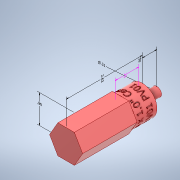
# Autodesk Inventor part: 1x8mmx1_1-inchHexShaft
Saved by Autodesk Inventor 2022.2 (Build 262287000, 287)
## iProperties
Created: 2020-11-16
Part Number: 1x8mmx1_1-inchHexShaft
Material: PC/ABS Plastic
Document SubType Name: Modeling
Designer: robst
Density: 0.357273 g/cm^3
Appearance: Smooth - Red
Author: robst
Autodesk Inventor part; units mm, degrees
ref_plane "XZ Plane" through (0, 0, 0) normal (0, 1, 0) x (-1, 0, 0)
ref_plane "XY Plane" through (0, 0, 0) normal (0, 0, 1) x (1, 0, 0)
sketch "Sketch1" plane through (0, 0, 0) normal (0, 0, 1) x (1, 0, 0)
  line L0 (14.6647, 0) -> (7.3323, -12.7)
  line L1 (7.3323, -12.7) -> (-7.3323, -12.7)
  line L2 (-7.3323, -12.7) -> (-14.6647, 0)
  line L3 (-14.6647, 0) -> (-7.3323, 12.7)
  line L4 (-7.3323, 12.7) -> (7.3323, 12.7)
  line L5 (7.3323, 12.7) -> (14.6647, 0)
  point P0 (0, 0)
  point P1 (0, 0)
  dimension "d0" = 25.4
  constraints: 12 end point, 1 coincident, 1 horizontal, 13 other
  measures "d0" distance between parallel lines of L1 L4
extrude "Hex Portion" add sketch "Sketch1" along normal mid plane 47.625
sketch "Sketch2" plane through (0, 0, -23.8125) normal (0, 0, -1) x (-1, 0, 0)
  circle A0 centre (0, 0) radius 12.7
  dimension "d3" = 25.4
  constraints: 1 centre point, 1 coincident
  measures "d3" diameter of A0
extrude "Extrusion2" add sketch "Sketch2" along normal blind 19.05
thicken "Reduce Size of Hex Shaft" operation add thickness 0.1905 both sides no extend neighbours yes toward (-0.8660254, -0.5, 0) faces at (10.9985, 6.35, 7.9375) (0, 12.7, 7.9375) (10.9985, -6.35, 7.9375) (0, -12.7, 7.9375) (-10.9985, -6.35, 7.9375) (-10.9985, 6.35, 7.9375)
sketch "Sketch3" plane through (0, 0, -42.8625) normal (0, 0, -1) x (-1, 0, 0)
  circle A0 centre (0, 0) radius 4
  dimension "d14" = 8
  constraints: 1 centre point, 1 coincident
  measures "d14" diameter of A0
extrude "Extrusion3" add sketch "Sketch3" along normal blind 12.7
ref_plane "Work Plane1" through (12.7, 0, -23.8125) normal (1, 0, 0) x (0, 1, 0)
sketch "Sketch4" plane through (12.7, 0, -23.8125) normal (1, 0, 0) x (0, 1, 0)
  line L0 (-12.7, 0) -> (12.7, 0) projected
  line L1 (-12.7, -19.05) -> (12.7, -19.05) projected
  line L2 (-12.7, 0) -> (-12.7, -19.05) construction
  line L3 (-12.7, -9.525) -> (12.7, -9.525) construction
  line L4 (12.7, 0) -> (12.7, -19.05) construction
  line L5 (-33.1661, -6.985) -> (-35.6444, -6.985)
  line L6 (-35.6444, -6.985) -> (-35.6444, -6.4663)
  line L7 (-35.6444, -6.4663) -> (-34.7223, -6.4663)
  line L8 (-34.7223, -6.4663) -> (-34.7223, -3.0618)
  line L9 (-34.7223, -3.0618) -> (-35.6444, -3.0618)
  line L10 (-35.6444, -3.0618) -> (-35.6444, -2.5966)
  spline S0 degree 2 poles (-35.6444, -2.5966) (-35.1216, -2.5966) (-34.6276, -2.3002) (-34.5946, -1.8885) knots 0 0 0 1 2 2 2
  line L11 (-34.5946, -1.8885) -> (-34.0677, -1.8885)
  line L12 (-34.0677, -1.8885) -> (-34.0677, -6.4663)
  line L13 (-34.0677, -6.4663) -> (-33.1661, -6.4663)
  line L14 (-33.1661, -6.4663) -> (-33.1661, -6.985)
  line L15 (-31.4701, -1.6786) -> (-31.6183, -3.6546)
  line L16 (-31.6183, -3.6546) -> (-32.067, -3.6546)
  line L17 (-32.067, -3.6546) -> (-32.2152, -1.6786)
  line L18 (-32.2152, -1.6786) -> (-31.4701, -1.6786)
  line L19 (-30.1857, -1.6786) -> (-30.3339, -3.6546)
  line L20 (-30.3339, -3.6546) -> (-30.7826, -3.6546)
  line L21 (-30.7826, -3.6546) -> (-30.9308, -1.6786)
  line L22 (-30.9308, -1.6786) -> (-30.1857, -1.6786)
  line L23 (-24.1918, -6.985) -> (-24.978, -6.985)
  line L24 (-24.978, -6.985) -> (-25.9043, -5.5524)
  line L25 (-25.9043, -5.5524) -> (-26.8553, -6.985)
  line L26 (-26.8553, -6.985) -> (-27.5839, -6.985)
  line L27 (-27.5839, -6.985) -> (-26.2624, -5.0954)
  line L28 (-26.2624, -5.0954) -> (-27.5716, -3.1729)
  line L29 (-27.5716, -3.1729) -> (-26.7853, -3.1729)
  line L30 (-26.7853, -3.1729) -> (-25.8631, -4.5932)
  line L31 (-25.8631, -4.5932) -> (-24.9204, -3.1729)
  line L32 (-24.9204, -3.1729) -> (-24.1918, -3.1729)
  line L33 (-24.1918, -3.1729) -> (-25.505, -5.0543)
  line L34 (-25.505, -5.0543) -> (-24.1918, -6.985)
  spline S1 degree 2 poles (-20.0709, -7.1003) (-20.4497, -7.1003) (-21.0713, -6.8738) (-21.2895, -6.6639) knots 0 0 0 1 2 2 2
  spline S2 degree 2 poles (-21.2895, -6.6639) (-21.5036, -6.4581) (-21.7259, -5.8982) (-21.7259, -5.5812) knots 0 0 0 1 2 2 2
  spline S3 degree 2 poles (-21.7259, -5.5812) (-21.7259, -5.1695) (-21.2854, -4.4779) (-20.8655, -4.2721) knots 0 0 0 1 2 2 2
  line L35 (-20.8655, -4.2721) -> (-20.8655, -4.2515)
  spline S4 degree 2 poles (-20.8655, -4.2515) (-21.2401, -4.0333) (-21.6024, -3.5146) (-21.6024, -3.1277) knots 0 0 0 1 2 2 2
  spline S5 degree 2 poles (-21.6024, -3.1277) (-21.6024, -2.5554) (-20.7378, -1.7897) (-20.0709, -1.7897) knots 0 0 0 1 2 2 2
  spline S6 degree 2 poles (-20.0709, -1.7897) (-19.3793, -1.7897) (-18.5436, -2.5143) (-18.5436, -3.0824) knots 0 0 0 1 2 2 2
  spline S7 degree 2 poles (-18.5436, -3.0824) (-18.5436, -3.4241) (-18.943, -4.091) (-19.3176, -4.2803) knots 0 0 0 1 2 2 2
  line L36 (-19.3176, -4.2803) -> (-19.3176, -4.3009)
  spline S8 degree 2 poles (-19.3176, -4.3009) (-18.873, -4.5068) (-18.416, -5.0996) (-18.416, -5.5689) knots 0 0 0 1 2 2 2
  spline S9 degree 2 poles (-18.416, -5.5689) (-18.416, -6.2193) (-19.3629, -7.1003) (-20.0709, -7.1003) knots 0 0 0 1 2 2 2
  spline S10 degree 2 poles (-19.1159, -5.6347) (-19.1159, -5.3219) (-19.3629, -4.9514) (-19.7128, -4.762) knots 0 0 0 1 2 2 2
  spline S11 degree 2 poles (-19.7128, -4.762) (-19.8281, -4.6961) (-20.215, -4.5438) (-20.4579, -4.445) knots 0 0 0 1 2 2 2
  spline S12 degree 2 poles (-20.4579, -4.445) (-20.7378, -4.6303) (-21.0384, -5.1819) (-21.0384, -5.5318) knots 0 0 0 1 2 2 2
  spline S13 degree 2 poles (-21.0384, -5.5318) (-21.0384, -5.9929) (-20.4826, -6.5939) (-20.0627, -6.5939) knots 0 0 0 1 2 2 2
  spline S14 degree 2 poles (-20.0627, -6.5939) (-19.6346, -6.5939) (-19.1159, -6.0793) (-19.1159, -5.6347) knots 0 0 0 1 2 2 2
  spline S15 degree 2 poles (-19.2106, -3.0906) (-19.2106, -2.7489) (-19.6675, -2.292) (-20.0751, -2.292) knots 0 0 0 1 2 2 2
  spline S16 degree 2 poles (-20.0751, -2.292) (-20.4456, -2.292) (-20.919, -2.6995) (-20.919, -3.0494) knots 0 0 0 1 2 2 2
  spline S17 degree 2 poles (-20.919, -3.0494) (-20.919, -3.3006) (-20.6761, -3.6505) (-20.4332, -3.7904) knots 0 0 0 1 2 2 2
  spline S18 degree 2 poles (-20.4332, -3.7904) (-20.3303, -3.8481) (-19.8939, -4.0498) (-19.7169, -4.1074) knots 0 0 0 1 2 2 2
  spline S19 degree 2 poles (-19.7169, -4.1074) (-19.4205, -3.881) (-19.2106, -3.3994) (-19.2106, -3.0906) knots 0 0 0 1 2 2 2
  line L37 (-13.3772, -6.985) -> (-13.3772, -4.7785)
  spline S20 degree 2 poles (-13.3772, -4.7785) (-13.3772, -4.515) (-13.4184, -4.0663) (-13.4842, -3.9428) knots 0 0 0 1 2 2 2
  spline S21 degree 2 poles (-13.4842, -3.9428) (-13.5501, -3.8069) (-13.8012, -3.6752) (-14.0194, -3.6752) knots 0 0 0 1 2 2 2
  spline S22 degree 2 poles (-14.0194, -3.6752) (-14.217, -3.6752) (-14.6698, -3.9181) (-14.9086, -4.1486) knots 0 0 0 1 2 2 2
  spline S23 degree 2 poles (-14.9086, -4.1486) (-14.9045, -4.2062) (-14.8963, -4.3668) (-14.8963, -4.4738) knots 0 0 0 1 2 2 2
  line L38 (-14.8963, -4.4738) -> (-14.8963, -6.985)
  line L39 (-14.8963, -6.985) -> (-15.5385, -6.985)
  line L40 (-15.5385, -6.985) -> (-15.5385, -4.7785)
  spline S24 degree 2 poles (-15.5385, -4.7785) (-15.5385, -4.515) (-15.5796, -4.0663) (-15.6455, -3.9428) knots 0 0 0 1 2 2 2
  spline S25 degree 2 poles (-15.6455, -3.9428) (-15.7114, -3.8069) (-15.9625, -3.6752) (-16.1807, -3.6752) knots 0 0 0 1 2 2 2
  spline S26 degree 2 poles (-16.1807, -3.6752) (-16.3865, -3.6752) (-16.8435, -3.9345) (-17.0575, -4.1362) knots 0 0 0 1 2 2 2
  line L41 (-17.0575, -4.1362) -> (-17.0575, -6.985)
  line L42 (-17.0575, -6.985) -> (-17.6997, -6.985)
  line L43 (-17.6997, -6.985) -> (-17.6997, -3.1729)
  line L44 (-17.6997, -3.1729) -> (-17.0575, -3.1729)
  line L45 (-17.0575, -3.1729) -> (-17.0575, -3.5928)
  spline S27 degree 2 poles (-17.0575, -3.5928) (-16.8064, -3.3417) (-16.3124, -3.0659) (-16.016, -3.0659) knots 0 0 0 1 2 2 2
  spline S28 degree 2 poles (-16.016, -3.0659) (-15.6784, -3.0659) (-15.1556, -3.3747) (-15.0198, -3.7246) knots 0 0 0 1 2 2 2
  spline S29 degree 2 poles (-15.0198, -3.7246) (-14.7275, -3.3994) (-14.1758, -3.0659) (-13.8547, -3.0659) knots 0 0 0 1 2 2 2
  spline S30 degree 2 poles (-13.8547, -3.0659) (-13.6077, -3.0659) (-13.2043, -3.2182) (-13.0561, -3.3911) knots 0 0 0 1 2 2 2
  spline S31 degree 2 poles (-13.0561, -3.3911) (-12.9038, -3.564) (-12.735, -4.0827) (-12.735, -4.4738) knots 0 0 0 1 2 2 2
  line L46 (-12.735, -4.4738) -> (-12.735, -6.985)
  line L47 (-12.735, -6.985) -> (-13.3772, -6.985)
  line L48 (-7.5109, -6.985) -> (-7.5109, -4.7785)
  spline S32 degree 2 poles (-7.5109, -4.7785) (-7.5109, -4.515) (-7.5521, -4.0663) (-7.6179, -3.9428) knots 0 0 0 1 2 2 2
  spline S33 degree 2 poles (-7.6179, -3.9428) (-7.6838, -3.8069) (-7.9349, -3.6752) (-8.1531, -3.6752) knots 0 0 0 1 2 2 2
  spline S34 degree 2 poles (-8.1531, -3.6752) (-8.3507, -3.6752) (-8.8036, -3.9181) (-9.0423, -4.1486) knots 0 0 0 1 2 2 2
  spline S35 degree 2 poles (-9.0423, -4.1486) (-9.0382, -4.2062) (-9.03, -4.3668) (-9.03, -4.4738) knots 0 0 0 1 2 2 2
  line L49 (-9.03, -4.4738) -> (-9.03, -6.985)
  line L50 (-9.03, -6.985) -> (-9.6722, -6.985)
  line L51 (-9.6722, -6.985) -> (-9.6722, -4.7785)
  spline S36 degree 2 poles (-9.6722, -4.7785) (-9.6722, -4.515) (-9.7133, -4.0663) (-9.7792, -3.9428) knots 0 0 0 1 2 2 2
  spline S37 degree 2 poles (-9.7792, -3.9428) (-9.8451, -3.8069) (-10.0962, -3.6752) (-10.3144, -3.6752) knots 0 0 0 1 2 2 2
  spline S38 degree 2 poles (-10.3144, -3.6752) (-10.5202, -3.6752) (-10.9772, -3.9345) (-11.1912, -4.1362) knots 0 0 0 1 2 2 2
  line L52 (-11.1912, -4.1362) -> (-11.1912, -6.985)
  line L53 (-11.1912, -6.985) -> (-11.8334, -6.985)
  line L54 (-11.8334, -6.985) -> (-11.8334, -3.1729)
  line L55 (-11.8334, -3.1729) -> (-11.1912, -3.1729)
  line L56 (-11.1912, -3.1729) -> (-11.1912, -3.5928)
  spline S39 degree 2 poles (-11.1912, -3.5928) (-10.9401, -3.3417) (-10.4461, -3.0659) (-10.1497, -3.0659) knots 0 0 0 1 2 2 2
  spline S40 degree 2 poles (-10.1497, -3.0659) (-9.8121, -3.0659) (-9.2893, -3.3747) (-9.1535, -3.7246) knots 0 0 0 1 2 2 2
  spline S41 degree 2 poles (-9.1535, -3.7246) (-8.8612, -3.3994) (-8.3095, -3.0659) (-7.9884, -3.0659) knots 0 0 0 1 2 2 2
  spline S42 degree 2 poles (-7.9884, -3.0659) (-7.7414, -3.0659) (-7.338, -3.2182) (-7.1898, -3.3911) knots 0 0 0 1 2 2 2
  spline S43 degree 2 poles (-7.1898, -3.3911) (-7.0375, -3.564) (-6.8687, -4.0827) (-6.8687, -4.4738) knots 0 0 0 1 2 2 2
  line L57 (-6.8687, -4.4738) -> (-6.8687, -6.985)
  line L58 (-6.8687, -6.985) -> (-7.5109, -6.985)
  line L59 (-0.8254, -6.985) -> (-1.6117, -6.985)
  line L60 (-1.6117, -6.985) -> (-2.5379, -5.5524)
  line L61 (-2.5379, -5.5524) -> (-3.4889, -6.985)
  line L62 (-3.4889, -6.985) -> (-4.2176, -6.985)
  line L63 (-4.2176, -6.985) -> (-2.8961, -5.0954)
  line L64 (-2.8961, -5.0954) -> (-4.2052, -3.1729)
  line L65 (-4.2052, -3.1729) -> (-3.4189, -3.1729)
  line L66 (-3.4189, -3.1729) -> (-2.4968, -4.5932)
  line L67 (-2.4968, -4.5932) -> (-1.5541, -3.1729)
  line L68 (-1.5541, -3.1729) -> (-0.8254, -3.1729)
  line L69 (-0.8254, -3.1729) -> (-2.1386, -5.0543)
  line L70 (-2.1386, -5.0543) -> (-0.8254, -6.985)
  line L71 (4.6375, -6.985) -> (2.1592, -6.985)
  line L72 (2.1592, -6.985) -> (2.1592, -6.4663)
  line L73 (2.1592, -6.4663) -> (3.0813, -6.4663)
  line L74 (3.0813, -6.4663) -> (3.0813, -3.0618)
  line L75 (3.0813, -3.0618) -> (2.1592, -3.0618)
  line L76 (2.1592, -3.0618) -> (2.1592, -2.5966)
  spline S44 degree 2 poles (2.1592, -2.5966) (2.682, -2.5966) (3.176, -2.3002) (3.209, -1.8885) knots 0 0 0 1 2 2 2
  line L77 (3.209, -1.8885) -> (3.7359, -1.8885)
  line L78 (3.7359, -1.8885) -> (3.7359, -6.4663)
  line L79 (3.7359, -6.4663) -> (4.6375, -6.4663)
  line L80 (4.6375, -6.4663) -> (4.6375, -6.985)
  line L81 (6.6629, -6.985) -> (5.8478, -6.985)
  line L82 (5.8478, -6.985) -> (5.8478, -6.0135)
  line L83 (5.8478, -6.0135) -> (6.6629, -6.0135)
  line L84 (6.6629, -6.0135) -> (6.6629, -6.985)
  spline S45 degree 2 poles (10.8495, -4.445) (10.8495, -5.8117) (10.055, -7.092) (9.2276, -7.092) knots 0 0 0 1 2 2 2
  spline S46 degree 2 poles (9.2276, -7.092) (8.3878, -7.092) (7.6015, -5.787) (7.6015, -4.4491) knots 0 0 0 1 2 2 2
  spline S47 degree 2 poles (7.6015, -4.4491) (7.6015, -3.0741) (8.396, -1.8021) (9.2276, -1.8021) knots 0 0 0 1 2 2 2
  spline S48 degree 2 poles (9.2276, -1.8021) (10.0633, -1.8021) (10.8495, -3.1194) (10.8495, -4.445) knots 0 0 0 1 2 2 2
  spline S49 degree 2 poles (9.9768, -5.9929) (10.0756, -5.7418) (10.1579, -4.9678) (10.1579, -4.445) knots 0 0 0 1 2 2 2
  spline S50 degree 2 poles (10.1579, -4.445) (10.1579, -3.9222) (10.0756, -3.1524) (9.9727, -2.893) knots 0 0 0 1 2 2 2
  spline S51 degree 2 poles (9.9727, -2.893) (9.8698, -2.6337) (9.5116, -2.3661) (9.2276, -2.3661) knots 0 0 0 1 2 2 2
  spline S52 degree 2 poles (9.2276, -2.3661) (8.9435, -2.3661) (8.5771, -2.6337) (8.4701, -2.9012) knots 0 0 0 1 2 2 2
  spline S53 degree 2 poles (8.4701, -2.9012) (8.3672, -3.1606) (8.2931, -3.951) (8.2931, -4.4491) knots 0 0 0 1 2 2 2
  spline S54 degree 2 poles (8.2931, -4.4491) (8.2931, -4.9843) (8.3589, -5.7006) (8.466, -5.9805) knots 0 0 0 1 2 2 2
  spline S55 degree 2 poles (8.466, -5.9805) (8.5648, -6.244) (8.9312, -6.528) (9.2276, -6.528) knots 0 0 0 1 2 2 2
  spline S56 degree 2 poles (9.2276, -6.528) (9.5075, -6.528) (9.8739, -6.2605) (9.9768, -5.9929) knots 0 0 0 1 2 2 2
  line L85 (12.2616, -1.6786) -> (12.1134, -3.6546)
  line L86 (12.1134, -3.6546) -> (11.6647, -3.6546)
  line L87 (11.6647, -3.6546) -> (11.5164, -1.6786)
  line L88 (11.5164, -1.6786) -> (12.2616, -1.6786)
  line L89 (13.546, -1.6786) -> (13.3978, -3.6546)
  line L90 (13.3978, -3.6546) -> (12.9491, -3.6546)
  line L91 (12.9491, -3.6546) -> (12.8009, -1.6786)
  line L92 (12.8009, -1.6786) -> (13.546, -1.6786)
  spline S57 degree 2 poles (18.6136, -7.0756) (18.1196, -7.0756) (17.2839, -6.7421) (16.9793, -6.4087) knots 0 0 0 1 2 2 2
  spline S58 degree 2 poles (16.9793, -6.4087) (16.6747, -6.0793) (16.3412, -5.0913) (16.3412, -4.4491) knots 0 0 0 1 2 2 2
  spline S59 degree 2 poles (16.3412, -4.4491) (16.3412, -3.811) (16.6664, -2.8642) (16.9752, -2.5143) knots 0 0 0 1 2 2 2
  spline S60 degree 2 poles (16.9752, -2.5143) (17.2798, -2.1726) (18.1114, -1.8144) (18.626, -1.8144) knots 0 0 0 1 2 2 2
  spline S61 degree 2 poles (18.626, -1.8144) (18.8812, -1.8144) (19.3299, -1.8885) (19.5193, -1.9462) knots 0 0 0 1 2 2 2
  spline S62 degree 2 poles (19.5193, -1.9462) (19.684, -1.9997) (20.0257, -2.152) (20.1944, -2.2426) knots 0 0 0 1 2 2 2
  line L93 (20.1944, -2.2426) -> (20.1944, -3.0577)
  line L94 (20.1944, -3.0577) -> (20.1409, -3.0577)
  spline S63 degree 2 poles (20.1409, -3.0577) (20.0504, -2.9753) (19.7704, -2.7448) (19.5687, -2.6337) knots 0 0 0 1 2 2 2
  spline S64 degree 2 poles (19.5687, -2.6337) (19.3752, -2.5266) (18.9183, -2.3908) (18.6219, -2.3908) knots 0 0 0 1 2 2 2
  spline S65 degree 2 poles (18.6219, -2.3908) (18.2966, -2.3908) (17.7162, -2.6584) (17.498, -2.9136) knots 0 0 0 1 2 2 2
  spline S66 degree 2 poles (17.498, -2.9136) (17.2839, -3.1729) (17.0452, -3.9592) (17.0452, -4.4491) knots 0 0 0 1 2 2 2
  spline S67 degree 2 poles (17.0452, -4.4491) (17.0452, -4.9719) (17.2963, -5.7253) (17.5145, -5.9846) knots 0 0 0 1 2 2 2
  spline S68 degree 2 poles (17.5145, -5.9846) (17.7285, -6.2358) (18.3008, -6.491) (18.6219, -6.491) knots 0 0 0 1 2 2 2
  spline S69 degree 2 poles (18.6219, -6.491) (18.9141, -6.491) (19.4123, -6.3469) (19.6058, -6.2399) knots 0 0 0 1 2 2 2
  spline S70 degree 2 poles (19.6058, -6.2399) (19.791, -6.1328) (20.0668, -5.9105) (20.145, -5.8323) knots 0 0 0 1 2 2 2
  line L95 (20.145, -5.8323) -> (20.1944, -5.8323)
  line L96 (20.1944, -5.8323) -> (20.1944, -6.6392)
  spline S71 degree 2 poles (20.1944, -6.6392) (20.0257, -6.7174) (19.7293, -6.8615) (19.5193, -6.9274) knots 0 0 0 1 2 2 2
  spline S72 degree 2 poles (19.5193, -6.9274) (19.297, -7.0015) (18.9183, -7.0756) (18.6136, -7.0756) knots 0 0 0 1 2 2 2
  spline S73 degree 2 poles (22.4298, -7.0715) (21.5159, -7.0715) (20.5114, -6.0464) (20.5114, -5.0996) knots 0 0 0 1 2 2 2
  spline S74 degree 2 poles (20.5114, -5.0996) (20.5114, -4.1692) (21.4871, -3.0659) (22.2734, -3.0659) knots 0 0 0 1 2 2 2
  spline S75 degree 2 poles (22.2734, -3.0659) (22.6274, -3.0659) (23.1749, -3.2717) (23.3766, -3.4899) knots 0 0 0 1 2 2 2
  spline S76 degree 2 poles (23.3766, -3.4899) (23.5825, -3.7081) (23.8007, -4.338) (23.8007, -4.7949) knots 0 0 0 1 2 2 2
  line L97 (23.8007, -4.7949) -> (23.8007, -5.1448)
  line L98 (23.8007, -5.1448) -> (21.1619, -5.1448)
  spline S77 degree 2 poles (21.1619, -5.1448) (21.1619, -5.8076) (21.8288, -6.5116) (22.4216, -6.5116) knots 0 0 0 1 2 2 2
  spline S78 degree 2 poles (22.4216, -6.5116) (22.6315, -6.5116) (23.0391, -6.4169) (23.2037, -6.3428) knots 0 0 0 1 2 2 2
  spline S79 degree 2 poles (23.2037, -6.3428) (23.3766, -6.2605) (23.6154, -6.1164) (23.6936, -6.0505) knots 0 0 0 1 2 2 2
  line L99 (23.6936, -6.0505) -> (23.7307, -6.0505)
  line L100 (23.7307, -6.0505) -> (23.7307, -6.7503)
  spline S80 degree 2 poles (23.7307, -6.7503) (23.6195, -6.7956) (23.282, -6.9274) (23.1502, -6.9644) knots 0 0 0 1 2 2 2
  spline S81 degree 2 poles (23.1502, -6.9644) (22.965, -7.0179) (22.6603, -7.0715) (22.4298, -7.0715) knots 0 0 0 1 2 2 2
  spline S82 degree 2 poles (23.1749, -4.655) (23.1667, -4.3956) (23.0597, -4.0169) (22.9567, -3.8892) knots 0 0 0 1 2 2 2
  spline S83 degree 2 poles (22.9567, -3.8892) (22.8456, -3.7452) (22.4957, -3.5928) (22.2363, -3.5928) knots 0 0 0 1 2 2 2
  spline S84 degree 2 poles (22.2363, -3.5928) (21.9811, -3.5928) (21.6229, -3.7452) (21.4747, -3.8934) knots 0 0 0 1 2 2 2
  spline S85 degree 2 poles (21.4747, -3.8934) (21.3306, -4.0457) (21.1824, -4.4121) (21.1619, -4.655) knots 0 0 0 1 2 2 2
  line L101 (21.1619, -4.655) -> (23.1749, -4.655)
  line L102 (27.4439, -6.985) -> (26.8017, -6.985)
  line L103 (26.8017, -6.985) -> (26.8017, -4.8114)
  spline S86 degree 2 poles (26.8017, -4.8114) (26.8017, -4.5479) (26.7523, -4.0951) (26.6782, -3.9592) knots 0 0 0 1 2 2 2
  spline S87 degree 2 poles (26.6782, -3.9592) (26.6, -3.8151) (26.3201, -3.6752) (26.0813, -3.6752) knots 0 0 0 1 2 2 2
  spline S88 degree 2 poles (26.0813, -3.6752) (25.8425, -3.6752) (25.3362, -3.9304) (25.0933, -4.1362) knots 0 0 0 1 2 2 2
  line L104 (25.0933, -4.1362) -> (25.0933, -6.985)
  line L105 (25.0933, -6.985) -> (24.4511, -6.985)
  line L106 (24.4511, -6.985) -> (24.4511, -3.1729)
  line L107 (24.4511, -3.1729) -> (25.0933, -3.1729)
  line L108 (25.0933, -3.1729) -> (25.0933, -3.597)
  spline S89 degree 2 poles (25.0933, -3.597) (25.3815, -3.3376) (25.9372, -3.0659) (26.2501, -3.0659) knots 0 0 0 1 2 2 2
  spline S90 degree 2 poles (26.2501, -3.0659) (26.81, -3.0659) (27.4439, -3.8069) (27.4439, -4.5109) knots 0 0 0 1 2 2 2
  line L109 (27.4439, -4.5109) -> (27.4439, -6.985)
  spline S91 degree 2 poles (29.4982, -7.0591) (28.9753, -7.0591) (28.3867, -6.4622) (28.3867, -5.8159) knots 0 0 0 1 2 2 2
  line L110 (28.3867, -5.8159) -> (28.3867, -3.704)
  line L111 (28.3867, -3.704) -> (27.9544, -3.704)
  line L112 (27.9544, -3.704) -> (27.9544, -3.1729)
  line L113 (27.9544, -3.1729) -> (28.3867, -3.1729)
  line L114 (28.3867, -3.1729) -> (28.3867, -2.0779)
  line L115 (28.3867, -2.0779) -> (29.0289, -2.0779)
  line L116 (29.0289, -2.0779) -> (29.0289, -3.1729)
  line L117 (29.0289, -3.1729) -> (30.2104, -3.1729)
  line L118 (30.2104, -3.1729) -> (30.2104, -3.704)
  line L119 (30.2104, -3.704) -> (29.0289, -3.704)
  line L120 (29.0289, -3.704) -> (29.0289, -5.5195)
  spline S92 degree 2 poles (29.0289, -5.5195) (29.0289, -5.8076) (29.0494, -6.1246) (29.1194, -6.2605) knots 0 0 0 1 2 2 2
  spline S93 degree 2 poles (29.1194, -6.2605) (29.1771, -6.3798) (29.4364, -6.4992) (29.6587, -6.4992) knots 0 0 0 1 2 2 2
  spline S94 degree 2 poles (29.6587, -6.4992) (29.8152, -6.4992) (30.1074, -6.4045) (30.1733, -6.3757) knots 0 0 0 1 2 2 2
  line L121 (30.1733, -6.3757) -> (30.2104, -6.3757)
  line L122 (30.2104, -6.3757) -> (30.2104, -6.9521)
  spline S95 degree 2 poles (30.2104, -6.9521) (30.0292, -7.0015) (29.6587, -7.0591) (29.4982, -7.0591) knots 0 0 0 1 2 2 2
  spline S96 degree 2 poles (32.3387, -7.0715) (31.4248, -7.0715) (30.4203, -6.0464) (30.4203, -5.0996) knots 0 0 0 1 2 2 2
  spline S97 degree 2 poles (30.4203, -5.0996) (30.4203, -4.1692) (31.396, -3.0659) (32.1823, -3.0659) knots 0 0 0 1 2 2 2
  spline S98 degree 2 poles (32.1823, -3.0659) (32.5363, -3.0659) (33.0838, -3.2717) (33.2855, -3.4899) knots 0 0 0 1 2 2 2
  spline S99 degree 2 poles (33.2855, -3.4899) (33.4914, -3.7081) (33.7095, -4.338) (33.7095, -4.7949) knots 0 0 0 1 2 2 2
  line L123 (33.7095, -4.7949) -> (33.7095, -5.1448)
  line L124 (33.7095, -5.1448) -> (31.0707, -5.1448)
  spline S100 degree 2 poles (31.0707, -5.1448) (31.0707, -5.8076) (31.7376, -6.5116) (32.3305, -6.5116) knots 0 0 0 1 2 2 2
  spline S101 degree 2 poles (32.3305, -6.5116) (32.5404, -6.5116) (32.948, -6.4169) (33.1126, -6.3428) knots 0 0 0 1 2 2 2
  spline S102 degree 2 poles (33.1126, -6.3428) (33.2855, -6.2605) (33.5243, -6.1164) (33.6025, -6.0505) knots 0 0 0 1 2 2 2
  line L125 (33.6025, -6.0505) -> (33.6396, -6.0505)
  line L126 (33.6396, -6.0505) -> (33.6396, -6.7503)
  spline S103 degree 2 poles (33.6396, -6.7503) (33.5284, -6.7956) (33.1908, -6.9274) (33.0591, -6.9644) knots 0 0 0 1 2 2 2
  spline S104 degree 2 poles (33.0591, -6.9644) (32.8739, -7.0179) (32.5692, -7.0715) (32.3387, -7.0715) knots 0 0 0 1 2 2 2
  spline S105 degree 2 poles (33.0838, -4.655) (33.0756, -4.3956) (32.9685, -4.0169) (32.8656, -3.8892) knots 0 0 0 1 2 2 2
  spline S106 degree 2 poles (32.8656, -3.8892) (32.7545, -3.7452) (32.4046, -3.5928) (32.1452, -3.5928) knots 0 0 0 1 2 2 2
  spline S107 degree 2 poles (32.1452, -3.5928) (31.89, -3.5928) (31.5318, -3.7452) (31.3836, -3.8934) knots 0 0 0 1 2 2 2
  spline S108 degree 2 poles (31.3836, -3.8934) (31.2395, -4.0457) (31.0913, -4.4121) (31.0707, -4.655) knots 0 0 0 1 2 2 2
  line L127 (31.0707, -4.655) -> (33.0838, -4.655)
  line L128 (36.3813, -3.8604) -> (36.3483, -3.8604)
  spline S109 degree 2 poles (36.3483, -3.8604) (36.2742, -3.8398) (36.1137, -3.8316) (36.0025, -3.8316) knots 0 0 0 1 2 2 2
  spline S110 degree 2 poles (36.0025, -3.8316) (35.7432, -3.8316) (35.2327, -4.058) (35.0022, -4.2803) knots 0 0 0 1 2 2 2
  line L129 (35.0022, -4.2803) -> (35.0022, -6.985)
  line L130 (35.0022, -6.985) -> (34.36, -6.985)
  line L131 (34.36, -6.985) -> (34.36, -3.1729)
  line L132 (34.36, -3.1729) -> (35.0022, -3.1729)
  line L133 (35.0022, -3.1729) -> (35.0022, -3.741)
  spline S111 degree 2 poles (35.0022, -3.741) (35.3521, -3.4282) (35.8749, -3.1729) (36.1219, -3.1729) knots 0 0 0 1 2 2 2
  spline S112 degree 2 poles (36.1219, -3.1729) (36.2207, -3.1729) (36.3195, -3.1812) (36.3813, -3.1935) knots 0 0 0 1 2 2 2
  line L134 (36.3813, -3.1935) -> (36.3813, -3.8604)
  spline S113 degree 2 poles (-21.979, -15.6168) (-22.5307, -15.6168) (-23.3046, -15.3863) (-23.6463, -15.2216) knots 0 0 0 1 2 2 2
  line L135 (-23.6463, -15.2216) -> (-23.6463, -14.3735)
  line L136 (-23.6463, -14.3735) -> (-23.5969, -14.3735)
  spline S114 degree 2 poles (-23.5969, -14.3735) (-23.2634, -14.6864) (-22.4195, -15.0322) (-22.0284, -15.0322) knots 0 0 0 1 2 2 2
  spline S115 degree 2 poles (-22.0284, -15.0322) (-21.4686, -15.0322) (-20.8963, -14.567) (-20.8963, -14.1842) knots 0 0 0 1 2 2 2
  spline S116 degree 2 poles (-20.8963, -14.1842) (-20.8963, -13.8795) (-21.1969, -13.5008) (-21.5221, -13.4061) knots 0 0 0 1 2 2 2
  spline S117 degree 2 poles (-21.5221, -13.4061) (-21.7567, -13.3403) (-22.1478, -13.2497) (-22.4401, -13.1756) knots 0 0 0 1 2 2 2
  spline S118 degree 2 poles (-22.4401, -13.1756) (-22.7036, -13.1056) (-23.1194, -12.8957) (-23.2799, -12.7269) knots 0 0 0 1 2 2 2
  spline S119 degree 2 poles (-23.2799, -12.7269) (-23.4363, -12.5581) (-23.6092, -12.1053) (-23.6092, -11.8088) knots 0 0 0 1 2 2 2
  spline S120 degree 2 poles (-23.6092, -11.8088) (-23.6092, -11.1913) (-22.6459, -10.3557) (-21.9008, -10.3557) knots 0 0 0 1 2 2 2
  spline S121 degree 2 poles (-21.9008, -10.3557) (-21.4727, -10.3557) (-20.7152, -10.5244) (-20.39, -10.685) knots 0 0 0 1 2 2 2
  line L137 (-20.39, -10.685) -> (-20.39, -11.4919)
  line L138 (-20.39, -11.4919) -> (-20.4394, -11.4919)
  spline S122 degree 2 poles (-20.4394, -11.4919) (-20.6823, -11.2696) (-21.4397, -10.9402) (-21.8555, -10.9402) knots 0 0 0 1 2 2 2
  spline S123 degree 2 poles (-21.8555, -10.9402) (-22.3248, -10.9402) (-22.9053, -11.3807) (-22.9053, -11.7389) knots 0 0 0 1 2 2 2
  spline S124 degree 2 poles (-22.9053, -11.7389) (-22.9053, -12.06) (-22.5636, -12.4428) (-22.2425, -12.5293) knots 0 0 0 1 2 2 2
  spline S125 degree 2 poles (-22.2425, -12.5293) (-22.0284, -12.5869) (-21.4068, -12.7351) (-21.201, -12.7969) knots 0 0 0 1 2 2 2
  spline S126 degree 2 poles (-21.201, -12.7969) (-20.6782, -12.9574) (-20.1924, -13.6037) (-20.1924, -14.0771) knots 0 0 0 1 2 2 2
  spline S127 degree 2 poles (-20.1924, -14.0771) (-20.1924, -14.3777) (-20.4353, -14.954) (-20.6535, -15.1557) knots 0 0 0 1 2 2 2
  spline S128 degree 2 poles (-20.6535, -15.1557) (-20.8963, -15.378) (-21.5138, -15.6168) (-21.979, -15.6168) knots 0 0 0 1 2 2 2
  line L139 (-16.5615, -15.5262) -> (-17.2037, -15.5262)
  line L140 (-17.2037, -15.5262) -> (-17.2037, -13.3526)
  spline S129 degree 2 poles (-17.2037, -13.3526) (-17.2037, -13.0891) (-17.2531, -12.6363) (-17.3272, -12.5005) knots 0 0 0 1 2 2 2
  spline S130 degree 2 poles (-17.3272, -12.5005) (-17.4054, -12.3564) (-17.6853, -12.2164) (-17.9241, -12.2164) knots 0 0 0 1 2 2 2
  spline S131 degree 2 poles (-17.9241, -12.2164) (-18.1629, -12.2164) (-18.6692, -12.4716) (-18.9121, -12.6775) knots 0 0 0 1 2 2 2
  line L141 (-18.9121, -12.6775) -> (-18.9121, -15.5262)
  line L142 (-18.9121, -15.5262) -> (-19.5543, -15.5262)
  line L143 (-19.5543, -15.5262) -> (-19.5543, -10.2198)
  line L144 (-19.5543, -10.2198) -> (-18.9121, -10.2198)
  line L145 (-18.9121, -10.2198) -> (-18.9121, -12.1382)
  spline S132 degree 2 poles (-18.9121, -12.1382) (-18.6239, -11.8788) (-18.0682, -11.6071) (-17.7553, -11.6071) knots 0 0 0 1 2 2 2
  spline S133 degree 2 poles (-17.7553, -11.6071) (-17.1954, -11.6071) (-16.5615, -12.3481) (-16.5615, -13.0521) knots 0 0 0 1 2 2 2
  line L146 (-16.5615, -13.0521) -> (-16.5615, -15.5262)
  spline S134 degree 2 poles (-13.5357, -15.1228) (-13.6139, -15.1804) (-13.8774, -15.3863) (-14.0009, -15.448) knots 0 0 0 1 2 2 2
  spline S135 degree 2 poles (-14.0009, -15.448) (-14.1697, -15.5386) (-14.4866, -15.6333) (-14.7748, -15.6333) knots 0 0 0 1 2 2 2
  spline S136 degree 2 poles (-14.7748, -15.6333) (-15.0095, -15.6333) (-15.4335, -15.4562) (-15.594, -15.2957) knots 0 0 0 1 2 2 2
  spline S137 degree 2 poles (-15.594, -15.2957) (-15.7464, -15.1393) (-15.9316, -14.6782) (-15.9316, -14.4229) knots 0 0 0 1 2 2 2
  spline S138 degree 2 poles (-15.9316, -14.4229) (-15.9316, -14.0277) (-15.5982, -13.4679) (-15.2359, -13.3073) knots 0 0 0 1 2 2 2
  spline S139 degree 2 poles (-15.2359, -13.3073) (-14.9148, -13.1591) (-14.042, -13.048) (-13.5357, -13.0192) knots 0 0 0 1 2 2 2
  line L147 (-13.5357, -13.0192) -> (-13.5357, -12.8957)
  spline S140 degree 2 poles (-13.5357, -12.8957) (-13.5357, -12.6734) (-13.6715, -12.3975) (-13.795, -12.3193) knots 0 0 0 1 2 2 2
  spline S141 degree 2 poles (-13.795, -12.3193) (-13.9185, -12.2411) (-14.2726, -12.1917) (-14.4619, -12.1917) knots 0 0 0 1 2 2 2
  spline S142 degree 2 poles (-14.4619, -12.1917) (-14.6842, -12.1917) (-15.2853, -12.3234) (-15.5858, -12.4511) knots 0 0 0 1 2 2 2
  line L148 (-15.5858, -12.4511) -> (-15.6229, -12.4511)
  line L149 (-15.6229, -12.4511) -> (-15.6229, -11.7965)
  spline S143 degree 2 poles (-15.6229, -11.7965) (-15.4458, -11.7471) (-14.783, -11.6236) (-14.4578, -11.6236) knots 0 0 0 1 2 2 2
  spline S144 degree 2 poles (-14.4578, -11.6236) (-14.0626, -11.6236) (-13.5233, -11.7471) (-13.3093, -11.9076) knots 0 0 0 1 2 2 2
  spline S145 degree 2 poles (-13.3093, -11.9076) (-13.0993, -12.0641) (-12.8935, -12.5622) (-12.8935, -12.9204) knots 0 0 0 1 2 2 2
  line L150 (-12.8935, -12.9204) -> (-12.8935, -15.5262)
  line L151 (-12.8935, -15.5262) -> (-13.5357, -15.5262)
  line L152 (-13.5357, -15.5262) -> (-13.5357, -15.1228)
  line L153 (-13.5357, -14.5876) -> (-13.5357, -13.5296)
  spline S146 degree 2 poles (-13.5357, -13.5296) (-13.7662, -13.5502) (-14.4619, -13.6202) (-14.6801, -13.6861) knots 0 0 0 1 2 2 2
  spline S147 degree 2 poles (-14.6801, -13.6861) (-14.9354, -13.7643) (-15.2688, -14.0895) (-15.2688, -14.3777) knots 0 0 0 1 2 2 2
  spline S148 degree 2 poles (-15.2688, -14.3777) (-15.2688, -14.707) (-14.8983, -15.0405) (-14.5443, -15.0405) knots 0 0 0 1 2 2 2
  spline S149 degree 2 poles (-14.5443, -15.0405) (-14.2438, -15.0405) (-13.7498, -14.7811) (-13.5357, -14.5876) knots 0 0 0 1 2 2 2
  line L154 (-9.9871, -10.8373) -> (-10.02, -10.8373)
  spline S150 degree 2 poles (-10.02, -10.8373) (-10.1065, -10.8044) (-10.4276, -10.7467) (-10.5552, -10.7467) knots 0 0 0 1 2 2 2
  spline S151 degree 2 poles (-10.5552, -10.7467) (-10.9586, -10.7467) (-11.3044, -11.109) (-11.3044, -11.5865) knots 0 0 0 1 2 2 2
  line L155 (-11.3044, -11.5865) -> (-11.3044, -11.7142)
  line L156 (-11.3044, -11.7142) -> (-10.2423, -11.7142)
  line L157 (-10.2423, -11.7142) -> (-10.2423, -12.2452)
  line L158 (-10.2423, -12.2452) -> (-11.2839, -12.2452)
  line L159 (-11.2839, -12.2452) -> (-11.2839, -15.5262)
  line L160 (-11.2839, -15.5262) -> (-11.9261, -15.5262)
  line L161 (-11.9261, -15.5262) -> (-11.9261, -12.2452)
  line L162 (-11.9261, -12.2452) -> (-12.3583, -12.2452)
  line L163 (-12.3583, -12.2452) -> (-12.3583, -11.7142)
  line L164 (-12.3583, -11.7142) -> (-11.9261, -11.7142)
  line L165 (-11.9261, -11.7142) -> (-11.9261, -11.5865)
  spline S152 degree 2 poles (-11.9261, -11.5865) (-11.9261, -10.9032) (-11.2633, -10.1869) (-10.6458, -10.1869) knots 0 0 0 1 2 2 2
  spline S153 degree 2 poles (-10.6458, -10.1869) (-10.4688, -10.1869) (-10.1271, -10.2239) (-9.9871, -10.2486) knots 0 0 0 1 2 2 2
  line L166 (-9.9871, -10.2486) -> (-9.9871, -10.8373)
  spline S154 degree 2 poles (-8.468, -15.6003) (-8.9909, -15.6003) (-9.5795, -15.0034) (-9.5795, -14.3571) knots 0 0 0 1 2 2 2
  line L167 (-9.5795, -14.3571) -> (-9.5795, -12.2452)
  line L168 (-9.5795, -12.2452) -> (-10.0118, -12.2452)
  line L169 (-10.0118, -12.2452) -> (-10.0118, -11.7142)
  line L170 (-10.0118, -11.7142) -> (-9.5795, -11.7142)
  line L171 (-9.5795, -11.7142) -> (-9.5795, -10.6191)
  line L172 (-9.5795, -10.6191) -> (-8.9373, -10.6191)
  line L173 (-8.9373, -10.6191) -> (-8.9373, -11.7142)
  line L174 (-8.9373, -11.7142) -> (-7.7559, -11.7142)
  line L175 (-7.7559, -11.7142) -> (-7.7559, -12.2452)
  line L176 (-7.7559, -12.2452) -> (-8.9373, -12.2452)
  line L177 (-8.9373, -12.2452) -> (-8.9373, -14.0607)
  spline S155 degree 2 poles (-8.9373, -14.0607) (-8.9373, -14.3488) (-8.9168, -14.6658) (-8.8468, -14.8017) knots 0 0 0 1 2 2 2
  spline S156 degree 2 poles (-8.8468, -14.8017) (-8.7891, -14.9211) (-8.5298, -15.0405) (-8.3075, -15.0405) knots 0 0 0 1 2 2 2
  spline S157 degree 2 poles (-8.3075, -15.0405) (-8.1511, -15.0405) (-7.8588, -14.9458) (-7.7929, -14.917) knots 0 0 0 1 2 2 2
  line L178 (-7.7929, -14.917) -> (-7.7559, -14.917)
  line L179 (-7.7559, -14.917) -> (-7.7559, -15.4933)
  spline S158 degree 2 poles (-7.7559, -15.4933) (-7.937, -15.5427) (-8.3075, -15.6003) (-8.468, -15.6003) knots 0 0 0 1 2 2 2
  line L180 (-1.3667, -10.4462) -> (-3.1163, -15.5262)
  line L181 (-3.1163, -15.5262) -> (-3.845, -15.5262)
  line L182 (-3.845, -15.5262) -> (-5.5946, -10.4462)
  line L183 (-5.5946, -10.4462) -> (-4.87, -10.4462)
  line L184 (-4.87, -10.4462) -> (-3.4621, -14.6658)
  line L185 (-3.4621, -14.6658) -> (-2.0542, -10.4462)
  line L186 (-2.0542, -10.4462) -> (-1.3667, -10.4462)
  spline S159 degree 2 poles (2.1942, -12.9862) (2.1942, -14.353) (1.3997, -15.6333) (0.5722, -15.6333) knots 0 0 0 1 2 2 2
  spline S160 degree 2 poles (0.5722, -15.6333) (-0.2676, -15.6333) (-1.0539, -14.3283) (-1.0539, -12.9903) knots 0 0 0 1 2 2 2
  spline S161 degree 2 poles (-1.0539, -12.9903) (-1.0539, -11.6154) (-0.2594, -10.3433) (0.5722, -10.3433) knots 0 0 0 1 2 2 2
  spline S162 degree 2 poles (0.5722, -10.3433) (1.4079, -10.3433) (2.1942, -11.6606) (2.1942, -12.9862) knots 0 0 0 1 2 2 2
  spline S163 degree 2 poles (1.3215, -14.5341) (1.4203, -14.283) (1.5026, -13.509) (1.5026, -12.9862) knots 0 0 0 1 2 2 2
  spline S164 degree 2 poles (1.5026, -12.9862) (1.5026, -12.4634) (1.4203, -11.6936) (1.3173, -11.4342) knots 0 0 0 1 2 2 2
  spline S165 degree 2 poles (1.3173, -11.4342) (1.2144, -11.1749) (0.8563, -10.9073) (0.5722, -10.9073) knots 0 0 0 1 2 2 2
  spline S166 degree 2 poles (0.5722, -10.9073) (0.2882, -10.9073) (-0.0782, -11.1749) (-0.1853, -11.4425) knots 0 0 0 1 2 2 2
  spline S167 degree 2 poles (-0.1853, -11.4425) (-0.2882, -11.7018) (-0.3623, -12.4922) (-0.3623, -12.9903) knots 0 0 0 1 2 2 2
  spline S168 degree 2 poles (-0.3623, -12.9903) (-0.3623, -13.5255) (-0.2964, -14.2418) (-0.1894, -14.5217) knots 0 0 0 1 2 2 2
  spline S169 degree 2 poles (-0.1894, -14.5217) (-0.0906, -14.7852) (0.2758, -15.0693) (0.5722, -15.0693) knots 0 0 0 1 2 2 2
  spline S170 degree 2 poles (0.5722, -15.0693) (0.8522, -15.0693) (1.2185, -14.8017) (1.3215, -14.5341) knots 0 0 0 1 2 2 2
  line L187 (5.7222, -15.5262) -> (3.244, -15.5262)
  line L188 (3.244, -15.5262) -> (3.244, -15.0075)
  line L189 (3.244, -15.0075) -> (4.1661, -15.0075)
  line L190 (4.1661, -15.0075) -> (4.1661, -11.603)
  line L191 (4.1661, -11.603) -> (3.244, -11.603)
  line L192 (3.244, -11.603) -> (3.244, -11.1378)
  spline S171 degree 2 poles (3.244, -11.1378) (3.7668, -11.1378) (4.2608, -10.8414) (4.2937, -10.4298) knots 0 0 0 1 2 2 2
  line L193 (4.2937, -10.4298) -> (4.8206, -10.4298)
  line L194 (4.8206, -10.4298) -> (4.8206, -15.0075)
  line L195 (4.8206, -15.0075) -> (5.7222, -15.0075)
  line L196 (5.7222, -15.0075) -> (5.7222, -15.5262)
  spline S172 degree 2 poles (12.1936, -11.9776) (12.1936, -12.307) (11.959, -12.8998) (11.749, -13.1056) knots 0 0 0 1 2 2 2
  spline S173 degree 2 poles (11.749, -13.1056) (11.4856, -13.365) (10.7734, -13.6325) (10.23, -13.6325) knots 0 0 0 1 2 2 2
  line L197 (10.23, -13.6325) -> (9.6578, -13.6325)
  line L198 (9.6578, -13.6325) -> (9.6578, -15.5262)
  line L199 (9.6578, -15.5262) -> (8.9826, -15.5262)
  line L200 (8.9826, -15.5262) -> (8.9826, -10.4462)
  line L201 (8.9826, -10.4462) -> (10.2588, -10.4462)
  spline S174 degree 2 poles (10.2588, -10.4462) (10.7116, -10.4462) (11.3456, -10.5944) (11.5885, -10.7632) knots 0 0 0 1 2 2 2
  spline S175 degree 2 poles (11.5885, -10.7632) (11.8725, -10.9567) (12.1936, -11.5536) (12.1936, -11.9776) knots 0 0 0 1 2 2 2
  spline S176 degree 2 poles (11.4897, -11.9982) (11.4897, -11.7347) (11.3086, -11.3478) (11.1233, -11.2243) knots 0 0 0 1 2 2 2
  spline S177 degree 2 poles (11.1233, -11.2243) (10.9628, -11.1172) (10.5346, -11.0308) (10.2176, -11.0308) knots 0 0 0 1 2 2 2
  line L202 (10.2176, -11.0308) -> (9.6578, -11.0308)
  line L203 (9.6578, -11.0308) -> (9.6578, -13.0562)
  line L204 (9.6578, -13.0562) -> (10.1188, -13.0562)
  spline S178 degree 2 poles (10.1188, -13.0562) (10.5305, -13.0562) (11.0369, -12.9245) (11.2015, -12.7516) knots 0 0 0 1 2 2 2
  spline S179 degree 2 poles (11.2015, -12.7516) (11.3538, -12.5993) (11.4897, -12.2411) (11.4897, -11.9982) knots 0 0 0 1 2 2 2
  line L205 (16.5203, -10.4462) -> (14.7707, -15.5262)
  line L206 (14.7707, -15.5262) -> (14.042, -15.5262)
  line L207 (14.042, -15.5262) -> (12.2924, -10.4462)
  line L208 (12.2924, -10.4462) -> (13.017, -10.4462)
  line L209 (13.017, -10.4462) -> (14.4249, -14.6658)
  line L210 (14.4249, -14.6658) -> (15.8328, -10.4462)
  line L211 (15.8328, -10.4462) -> (16.5203, -10.4462)
  spline S180 degree 2 poles (20.0812, -12.9862) (20.0812, -14.353) (19.2867, -15.6333) (18.4593, -15.6333) knots 0 0 0 1 2 2 2
  spline S181 degree 2 poles (18.4593, -15.6333) (17.6194, -15.6333) (16.8332, -14.3283) (16.8332, -12.9903) knots 0 0 0 1 2 2 2
  spline S182 degree 2 poles (16.8332, -12.9903) (16.8332, -11.6154) (17.6277, -10.3433) (18.4593, -10.3433) knots 0 0 0 1 2 2 2
  spline S183 degree 2 poles (18.4593, -10.3433) (19.2949, -10.3433) (20.0812, -11.6606) (20.0812, -12.9862) knots 0 0 0 1 2 2 2
  spline S184 degree 2 poles (19.2085, -14.5341) (19.3073, -14.283) (19.3896, -13.509) (19.3896, -12.9862) knots 0 0 0 1 2 2 2
  spline S185 degree 2 poles (19.3896, -12.9862) (19.3896, -12.4634) (19.3073, -11.6936) (19.2044, -11.4342) knots 0 0 0 1 2 2 2
  spline S186 degree 2 poles (19.2044, -11.4342) (19.1015, -11.1749) (18.7433, -10.9073) (18.4593, -10.9073) knots 0 0 0 1 2 2 2
  spline S187 degree 2 poles (18.4593, -10.9073) (18.1752, -10.9073) (17.8088, -11.1749) (17.7018, -11.4425) knots 0 0 0 1 2 2 2
  spline S188 degree 2 poles (17.7018, -11.4425) (17.5989, -11.7018) (17.5248, -12.4922) (17.5248, -12.9903) knots 0 0 0 1 2 2 2
  spline S189 degree 2 poles (17.5248, -12.9903) (17.5248, -13.5255) (17.5906, -14.2418) (17.6977, -14.5217) knots 0 0 0 1 2 2 2
  spline S190 degree 2 poles (17.6977, -14.5217) (17.7965, -14.7852) (18.1629, -15.0693) (18.4593, -15.0693) knots 0 0 0 1 2 2 2
  spline S191 degree 2 poles (18.4593, -15.0693) (18.7392, -15.0693) (19.1056, -14.8017) (19.2085, -14.5341) knots 0 0 0 1 2 2 2
  line L212 (23.6092, -15.5262) -> (21.131, -15.5262)
  line L213 (21.131, -15.5262) -> (21.131, -15.0075)
  line L214 (21.131, -15.0075) -> (22.0531, -15.0075)
  line L215 (22.0531, -15.0075) -> (22.0531, -11.603)
  line L216 (22.0531, -11.603) -> (21.131, -11.603)
  line L217 (21.131, -11.603) -> (21.131, -11.1378)
  spline S192 degree 2 poles (21.131, -11.1378) (21.6538, -11.1378) (22.1478, -10.8414) (22.1807, -10.4298) knots 0 0 0 1 2 2 2
  line L218 (22.1807, -10.4298) -> (22.7077, -10.4298)
  line L219 (22.7077, -10.4298) -> (22.7077, -15.0075)
  line L220 (22.7077, -15.0075) -> (23.6092, -15.0075)
  line L221 (23.6092, -15.0075) -> (23.6092, -15.5262)
  point P0 (0, 23.8125)
  constraints: 2 end point, 2 midpoint, 1 horizontal
emboss "Emboss1" sketch "Sketch4" operation cut depth 2.54 direction (-1, 0, 0) wrap yes faces at (-12.6095, -1.5136, -36.5125)
equation "\"d0\" = hexSize"
equation "\"d1\" = length"
equation "\"d6\" = printOffset"
equation "\"hexSize\" = 25.4"
equation "\"length\" = 47.625"
equation "\"printOffset\" = 0.1905"
body "Solid1"
